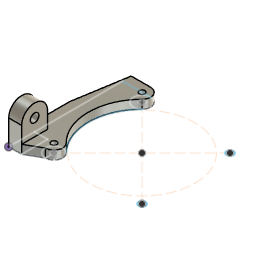
M60_BRACKET_A (Autodesk Fusion 360 design; units mm, degrees)
Autodesk Fusion 360 part; units mm, degrees
note: some values were not read from the file. Set by a fixed rule: which sketch regions a step uses.
sketch "Esquisse1" plane through (0, 0, 0) normal (0, 0, 1) x (1, 0, 0)
  circle A0 centre (16.25, 10) radius 1.65
  circle A1 centre (16.25, 61) radius 1.65
  circle A2 centre (67.25, 10) radius 1.95
  circle A3 centre (67.25, 61) radius 1.95
  line L0 (67.25, 61) -> (16.25, 10) construction
  line L1 (16.25, 61) -> (67.25, 10) construction
  circle A4 centre (41.75, 35.5) radius 30.5 construction
  circle A5 centre (16.25, 61) radius 5
  circle A6 centre (16.25, 10) radius 5
  arc A7 (19.7855, 57.4645) -> (19.7855, 13.5355) centre (41.75, 35.5) ccw
  line L2 (16.5063, 65.9934) -> (0, 65.9934)
  line L3 (0, 65.9934) -> (0, 0)
  line L4 (0, 0) -> (7.5, 0)
  line L5 (16.25, 10) -> (16.25, 5)
  line L6 (16.25, 5) -> (7.5, 0)
  line L7 (7.5, 0) -> (7.5, 15)
  line L8 (7.5, 15) -> (0, 15)
  dimension "d1" = 3.3
  dimension "d2" = 3.3
  dimension "d3" = 16.25
  dimension "d4" = 16.25
  dimension "d5" = 51
  dimension "d6" = 10
  dimension "d7" = 3.9
  dimension "d8" = 51
  dimension "d9" = 3.9
  dimension "d10" = 51
  dimension "d11" = 51
  dimension "d12" = 61
  dimension "d13" = 10
  dimension "d14" = 10
  dimension "d15" = 7.5
  dimension "d16" = 15
  constraint coincident A3.centre L0.start
  constraint coincident A0.centre L0.end
  constraint coincident A1.centre L1.start
  constraint coincident A2.centre L1.end
  constraint midpoint L0 A4.centre
  constraint concentric A1 A5
  constraint concentric A0 A6
  constraint coincident L1 A7.start
  constraint coincident A6 A7.end
  constraint coincident L0 A7.end
  constraint coincident A4.centre A7.centre
  constraint coincident A5 L2.start
  constraint horizontal L2
  constraint coincident L3.end L4.start
  constraint perpendicular L2 L3
  constraint perpendicular L3 L4
  constraint coincident A6 L5.end
  constraint vertical L5
  constraint perpendicular L4 L7
  constraint coincident L3 L8.end
  constraint perpendicular L3 L8
  measures "d1" diameter of A0
  measures "d2" diameter of A1
  measures "d3" horizontal distance of L3.end A0.centre
  measures "d4" horizontal distance of L3.end A1.centre
  measures "d5" distance of A0.centre A1.centre
  measures "d6" vertical distance of L3.end A0.centre
  measures "d7" diameter of A2
  measures "d8" distance of A0.centre A2.centre
  measures "d9" diameter of A3
  measures "d10" horizontal distance of A1.centre A3.centre
  measures "d11" distance of A2.centre A3.centre
  measures "d12" diameter of A4
  measures "d13" diameter of A5
  measures "d14" diameter of A6
  measures "d15" distance of L3.end L4.end
  measures "d16" distance of L4.end L7.end
extrude "Extrusion1" add sketch "Esquisse1" along normal blind 22 contours L3 L4 L7 L8 makes body 1
extrude "Extrusion2" add sketch "Esquisse1" along normal blind 5 separate body contours A5 L2 | A5 A6 A7 L2 L3 L6 L7 L8 | A6 picked at (18.7618, 58.051) makes body 2
sketch "Esquisse2" plane through (0, 0, 0) normal (-1, 0, 0) x (0, -1, 0)
  line L0 (-15, 0) -> (0, 0)
  line L1 (0, 0) -> (0, 22)
  line L2 (0, 22) -> (-15, 22)
  line L3 (-15, 22) -> (-15, 0)
  circle A0 centre (-7.5, 14.5) radius 2.5
  arc A1 (0, 14.5) -> (-7.5, 22) centre (-7.5, 14.5) ccw
  arc A2 (-7.5, 22) -> (-15, 14.5) centre (-7.5, 14.5) ccw
  dimension "d21" = 5
  dimension "d22" = 7.5
  dimension "d23" = 7.5
  constraint coincident L2 A1.end
  constraint coincident L1 A1.start
  constraint coincident A0.centre A1.centre
  constraint coincident L3 A2.end
  measures "d21" diameter of A0
  measures "d22" distance of L3 A0.centre
  measures "d23" distance of L2 A0.centre
extrude "Extrusion3" cut sketch "Esquisse2" against normal blind 8 contours L2 L3 A2 | L1 L2 A1 | A0 bodies 1
sketch "Esquisse3" plane through (0, 0, 5) normal (0, 0, 1) x (-1, 0, 0)
  circle A0 centre (-16.25, -61) radius 1.65
  circle A1 centre (-16.25, -10) radius 1.65
  arc A2 (-16.25, -5) -> (-19.7855, -13.5355) centre (-16.25, -10) ccw
  arc A3 (-19.7855, -57.4645) -> (-19.7855, -13.5355) centre (-41.75, -35.5) ccw
  arc A4 (-19.7855, -57.4645) -> (-16.5063, -65.9934) centre (-16.25, -61) ccw
  line L0 (-16.5063, -65.9934) -> (0, -65.9934)
  line L1 (0, -65.9934) -> (0, -15)
  line L2 (0, -15) -> (-7.5, -15)
  line L3 (-7.5, -15) -> (-7.5, 0)
  line L4 (-7.5, 0) -> (-16.25, -5)
  line L5 (0, -35.5) -> (-5, -66.0689)
  line L6 (-5, -66.0689) -> (0, -65.9934)
  line L7 (0, -35.5) -> (0, -65.9934)
  dimension "d27" = 5
  constraint coincident L1 L5.start
  constraint coincident L0.end L1.start
  measures "d27" horizontal distance of L5.end L0.end
extrude "Extrusion4" cut sketch "Esquisse3" against normal blind 10 contours L0 L1 L5 L7 bodies 2
combine "Combiner1" operation add target body 2 tool bodies 1
equation "d3 = 14.3 mm + 1.95 mm"
